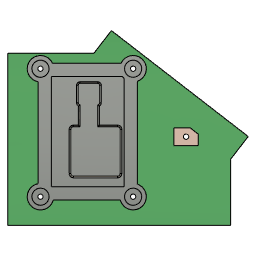
wiiWaterCooler_Base (Autodesk Fusion 360 design; units mm, degrees)
Autodesk Fusion 360 part; units mm, degrees
sketch "Wii" plane through (0, 0, 0) normal (0, 0, 1) x (1, 0, 0)
  line L0 (-39.75, -33.5) -> (61.25, -33.5)
  line L1 (-39.75, 44.5) -> (-39.75, -33.5)
  line L2 (-0.75, 44.5) -> (61.25, -3.5)
  line L3 (61.25, -33.5) -> (61.25, -3.5)
  line L4 (-39.75, 44.5) -> (-0.75, 44.5)
  circle A0 centre (-24.95, -20.5) radius 1.2
  circle A1 centre (-24.95, -20.5) radius 3.9
  circle A2 centre (41.05, 6.675) radius 1.2
  line L5 (14.5, -14.5) -> (-14.5, -14.5)
  line L6 (-14.5, -14.5) -> (-14.5, 14.5)
  line L7 (-14.5, 14.5) -> (14.5, 14.5)
  line L8 (14.5, 14.5) -> (14.5, -14.5)
  line L9 (14.5, -14.5) -> (-14.5, 14.5) construction
  line L10 (-14.5, -14.5) -> (14.5, 14.5) construction
  line L11 (4.5, 18.5) -> (-10.5, 18.5)
  line L12 (-10.5, 18.5) -> (-10.5, 33.5)
  line L13 (-10.5, 33.5) -> (4.5, 33.5)
  line L14 (4.5, 33.5) -> (4.5, 18.5)
  line L15 (4.5, 18.5) -> (-10.5, 33.5) construction
  line L16 (-10.5, 18.5) -> (4.5, 33.5) construction
  line L17 (10, 12.5) -> (-10, 12.5)
  line L18 (-12.5, 10) -> (-12.5, -10)
  line L19 (-10, -12.5) -> (10, -12.5)
  line L20 (12.5, -10) -> (12.5, 10)
  line L21 (12.5, 12.5) -> (-12.5, -12.5) construction
  line L22 (-12.5, 12.5) -> (12.5, -12.5) construction
  line L23 (1, 31.5) -> (-7, 31.5)
  line L24 (-8.5, 30) -> (-8.5, 22)
  line L25 (-7, 20.5) -> (1, 20.5)
  line L26 (2.5, 22) -> (2.5, 30)
  line L27 (2.5, 31.5) -> (-8.5, 20.5) construction
  line L28 (-8.5, 31.5) -> (2.5, 20.5) construction
  arc A3 (12.5, 10) -> (10, 12.5) centre (10, 10) ccw
  arc A4 (-10, 12.5) -> (-12.5, 10) centre (-10, 10) ccw
  arc A5 (-12.5, -10) -> (-10, -12.5) centre (-10, -10) ccw
  arc A6 (10, -12.5) -> (12.5, -10) centre (10, -10) ccw
  arc A7 (2.5, 30) -> (1, 31.5) centre (1, 30) ccw
  arc A8 (-7, 31.5) -> (-8.5, 30) centre (-7, 30) ccw
  arc A9 (-8.5, 22) -> (-7, 20.5) centre (-7, 22) ccw
  arc A10 (1, 20.5) -> (2.5, 22) centre (1, 22) ccw
  circle A11 centre (-24.95, 37.5) radius 1.2
  circle A12 centre (-24.95, 37.5) radius 3.9
  circle A13 centre (17.05, -20.5) radius 1.2
  circle A14 centre (17.05, -20.5) radius 3.9
  line L29 (42.9406, 10.675) -> (35.55, 10.675)
  line L30 (35.55, 10.675) -> (35.55, 2.675)
  line L31 (35.55, 2.675) -> (46.55, 2.675)
  line L32 (46.55, 2.675) -> (46.55, 7.8806)
  line L33 (44.6889, 9.3215) -> (35.55, 2.675) construction
  line L34 (35.55, 10.675) -> (46.55, 2.675) construction
  point P0 (-24.95, -20.5)
  point P1 (-3, 26)
  point P2 (41.05, 6.675)
  point P3 (-3, 26)
  point P4 (41.05, 6.675)
  dimension "d8" = 2.4
  dimension "d9" = 7.8
  dimension "d18" = 2.4
  dimension "d19" = 29
  dimension "d20" = 29
  dimension "d21" = 15
  dimension "d22" = 15
  dimension "d25" = 4
  dimension "d29" = 25
  dimension "d30" = 11
  dimension "d31" = 11
  dimension "d42" = 2.5
  dimension "d43" = 2.5
  dimension "d44" = 2.5
  dimension "d45" = 2.5
  dimension "d49" = 1.5
  dimension "d50" = 1.5
  dimension "d51" = 1.5
  dimension "d52" = 1.5
  dimension "d67" = 2.4
  dimension "d68" = 7.8
  dimension "d70" = 2.4
  dimension "d71" = 7.8
  constraint coincident P0 A0.centre
  constraint concentric A0 A1
  constraint perpendicular L5 L6
  constraint parallel L5 L7
  constraint parallel L6 L8
  constraint horizontal L5
  constraint coincident L9 origin
  constraint coincident L10 origin
  constraint perpendicular L11 L12
  constraint parallel L11 L13
  constraint parallel L12 L14
  constraint horizontal L11
  constraint coincident L15 P3
  constraint coincident L16 P3
  constraint coincident P4 P2
  constraint perpendicular L17 L18
  constraint parallel L17 L19
  constraint parallel L18 L20
  constraint horizontal L17
  constraint coincident L21 origin
  constraint coincident L22 origin
  constraint perpendicular L23 L24
  constraint parallel L23 L25
  constraint parallel L24 L26
  constraint horizontal L23
  constraint coincident L27 P3
  constraint coincident L28 P3
  constraint coincident P3 P1
  constraint tangent L20 A3
  constraint tangent L17 A3
  constraint tangent L18 A4
  constraint tangent L17 A4
  constraint coincident L21.end L19
  constraint coincident L21.end L18
  constraint tangent L19 A5
  constraint tangent L18 A5
  constraint coincident L22.end L19
  constraint coincident L22.end L20
  constraint tangent L19 A6
  constraint tangent L20 A6
  constraint tangent L26 A7
  constraint tangent L23 A7
  constraint coincident L28.start L24
  constraint coincident L28.start L23
  constraint tangent L24 A8
  constraint tangent L23 A8
  constraint coincident L27.end L25
  constraint coincident L27.end L24
  constraint tangent L25 A9
  constraint tangent L24 A9
  constraint coincident L28.end L25
  constraint coincident L28.end L26
  constraint tangent L25 A10
  constraint tangent L26 A10
  constraint concentric A11 A12
  constraint concentric A13 A14
  constraint perpendicular L29 L30
  constraint parallel L29 L31
  constraint parallel L30 L32
  constraint horizontal L29
  constraint coincident L33 P4
  constraint coincident L34 P4
  constraint coincident L2 L32.end
  constraint coincident L2 L33.start
  constraint coincident L2 L29.start
  measures "d8" diameter of A0
  measures "d9" diameter of A1
  measures "d18" diameter of A2
  measures "d19" distance of L6.end L7.end
  measures "d20" distance of L5.end L6.end
  measures "d21" distance of L12.end L13.end
  measures "d22" distance of L11.end L12.end
  measures "d25" distance of L7 L11
  measures "d29" distance of L21.end L22.end
  measures "d30" distance of L28.start L27.end
  measures "d31" distance of L27.end L28.end
  measures "d42" radius of A3
  measures "d43" radius of A4
  measures "d44" radius of A5
  measures "d45" radius of A6
  measures "d49" radius of A7
  measures "d50" radius of A8
  measures "d51" radius of A9
  measures "d52" radius of A10
  measures "d67" diameter of A11
  measures "d68" diameter of A12
  measures "d70" diameter of A13
  measures "d71" diameter of A14
extrude "Extrude14" add sketch "Wii" along normal blind 1.35 contours L2 L29 L30 L31 L32 | A1 | A12 | A14 makes body 1 at (-21.969, -20.7534, 0) makes body 2 at (20.031, -20.7534, 0) makes body 3 at (-21.969, 37.2466, 0) makes body 4 at (36.9833, 6.675, 0)
extrude "Extrude15" add sketch "Wii" along normal blind 1.35 separate body contours L0 L1 L2 L3 L4 L29 L30 L31 L32 | L5 L6 L7 L8 | L11 L12 L13 L14 | L17 L18 L19 L20 A3 A4 A5 A6 | L23 L24 L25 L26 A7 A8 A9 A10 makes body 5
extrude "Extrude16" add sketch "Wii" along normal blind 2 from surface at 1.35 separate body contours L5 L6 L7 L8 makes body 6
extrude "Extrude17" add sketch "Wii" along normal blind 2.75 from surface at 1.35 separate body contours L17 L18 L19 L20 A3 A4 A5 A6 makes body 7
combine "Combine4" operation add target body 7 tool bodies 6
fillet "Fillet3" radius 1.5 8 edges at (0, 12.5, 4.1) (-11.7678, 11.7678, 4.1) (-12.5, 0, 4.1) (-11.7678, -11.7678, 4.1) (0, -12.5, 4.1) (11.7678, -11.7678, 4.1) (12.5, 0, 4.1) (11.7678, 11.7678, 4.1) on bodies 7
extrude "Extrude18" add sketch "Wii" along normal blind 1.9 from surface at 1.35 separate body contours L11 L12 L13 L14 makes body 8
extrude "Extrude19" add sketch "Wii" along normal blind 2.65 from surface at 1.35 separate body contours L23 L24 L25 L26 A7 A8 A9 A10 makes body 9
combine "Combine5" operation add target body 9 tool bodies 8
fillet "Fillet4" radius 0.65 8 edges at (-3, 31.5, 4) (-8.0607, 31.0607, 4) (-8.5, 26, 4) (-8.0607, 20.9393, 4) (-3, 20.5, 4) (2.0607, 20.9393, 4) (2.5, 26, 4) (2.0607, 31.0607, 4) on bodies 9
copy_body "CopyPasteBodies1" bodies 1 makes body 10
move_body "Move1" bodies 10 to x (1, 0, 0) y (0, 1, 0) z (0, 0, 1) at (44, 58, 0)
move_body "Move3" bodies 10 to x (1, 0, 0) y (0, 1, 0) z (0, 0, 1) at (-2, 0, 0)
extrude "Extrude20" add 2 faces at (13.8135, 33.225, 0.45) (51.45, 4.0871, 0.9) along direction (0.612173, 0.790724, 0) blind 13 on bodies 5 bodies 5
extrude "Extrude21" add 1 faces at (45.5934, 14.1015, 0.45) along direction (0.790724, -0.612173, 0) blind 5 on bodies 5 bodies 5
sketch "Sketch2" plane through (0, 0, 1.35) normal (0, 0, 1) x (1, 0, 0)
  line L0 (46.55, 7.8806) -> (46.55, 2.675)
  line L1 (46.55, 2.675) -> (35.55, 2.675)
  line L2 (35.55, 2.675) -> (35.55, 10.675)
  line L3 (35.55, 10.675) -> (42.9406, 10.675)
  line L4 (42.9406, 10.675) -> (46.55, 7.8806)
  line L5 (69.2083, 6.7794) -> (7.2083, 54.7794)
  line L6 (7.2083, 54.7794) -> (-0.75, 44.5)
  line L7 (-0.75, 44.5) -> (-39.75, 44.5)
  line L8 (-39.75, 44.5) -> (-39.75, -33.5)
  line L9 (-39.75, -33.5) -> (61.25, -33.5)
  line L10 (61.25, -33.5) -> (61.25, -3.5)
  line L11 (61.25, -3.5) -> (69.2083, 6.7794)
  circle A0 centre (-24.95, 37.5) radius 3.9
  circle A1 centre (-24.95, -20.5) radius 3.9
  circle A2 centre (17.05, -20.5) radius 3.9
  circle A3 centre (17.05, 37.5) radius 1.1931
sketch "Sketch3" plane through (0, 0, 1.35) normal (0, 0, 1) x (1, 0, 0)
  circle A0 centre (17.05, 37.5) radius 3.8694
extrude "Extrude22" cut sketch "Sketch3" against normal blind 2 bodies 5
sketch "Sketch4" plane through (0, 0, 0) normal (0, 0, 1) x (1, 0, 0)
sketch "GPUcontact" plane through (0, 0, 4.1) normal (0, 0, 1) x (1, 0, 0)
  line L0 (11.201, -10) -> (11.201, 10)
  arc A0 (11.201, 10) -> (10, 11.201) centre (10, 10) ccw
  line L1 (10, 11.201) -> (-10, 11.201)
  arc A1 (-10, 11.201) -> (-11.201, 10) centre (-10, 10) ccw
  line L2 (-11.201, 10) -> (-11.201, -10)
  arc A2 (-11.201, -10) -> (-10, -11.201) centre (-10, -10) ccw
  line L3 (-10, -11.201) -> (10, -11.201)
  arc A3 (10, -11.201) -> (11.201, -10) centre (10, -10) ccw
sketch "CPUcontact" plane through (0, 0, 4) normal (0, 0, 1) x (1, 0, 0)
  line L0 (1, 30.85) -> (-7, 30.85)
  arc A0 (-7, 30.85) -> (-7.85, 30) centre (-7, 30) ccw
  line L1 (-7.85, 30) -> (-7.85, 22)
  arc A1 (-7.85, 22) -> (-7, 21.15) centre (-7, 22) ccw
  line L2 (-7, 21.15) -> (1, 21.15)
  arc A2 (1, 21.15) -> (1.85, 22) centre (1, 22) ccw
  line L3 (1.85, 22) -> (1.85, 30)
  arc A3 (1.85, 30) -> (1, 30.85) centre (1, 30) ccw
sketch "screwPost" plane through (0, 0, 1.35) normal (0, 0, 1) x (1, 0, 0)
  circle A0 centre (-24.95, 37.5) radius 1.2
  circle A1 centre (-24.95, 37.5) radius 3.9
extrude "Extrude23" add sketch "screwPost" 3 faces at (20.031, 37.2466, 1.35) (20.031, -20.7534, 1.35) (-21.969, -20.7534, 1.35) along normal blind 2.75 separate body on bodies 1 2 10 makes body 11 at (20.9452, -20.6944, 3.1833) makes body 12 at (-21.0548, 37.3056, 3.1833) makes body 13 at (20.9452, 37.3056, 3.1833) makes body 14 at (-21.0548, -20.6944, 3.1833)
extrude "Extrude24" add sketch "GPUcontact" along normal blind 3 separate body makes body 15
extrude "Extrude25" add sketch "CPUcontact" along normal blind 3.1 separate body makes body 16
extrude "Extrude26" add 4 faces at (-21.969, 37.2466, 4.1) (20.031, 37.2466, 4.1) (-21.969, -20.7534, 4.1) (20.031, -20.7534, 4.1) along direction (0, 0, 1) blind 3 on bodies 11 12 13 14 bodies 12 11 13 14
sketch "Sketch12" plane through (0, 0, 7.1) normal (0, 0, 1) x (1, 0, 0)
  circle A0 centre (-24.95, -20.5) radius 1.2
  circle A1 centre (-24.95, -20.5) radius 3.9
  line L0 (-24, -19) -> (16, -19)
  line L1 (16, -19) -> (16, 36)
  line L2 (16, 36) -> (-24, 36)
  line L3 (-24, 36) -> (-24, -19)
  line L4 (-20, -16) -> (13, -16)
  line L5 (13, -16) -> (13, 34)
  line L6 (13, 34) -> (-20, 34)
  line L7 (-20, 34) -> (-20, -16)
  constraint horizontal L0
  constraint vertical L1
  constraint horizontal L2
  constraint vertical L3
  constraint horizontal L4
  constraint vertical L5
  constraint horizontal L6
  constraint vertical L7
extrude "Extrude27" add sketch "Sketch12" along normal blind 2 separate body contours A1 L0 L3 | A1 L0 L1 L2 L3 picked at (-23.2156, -17.8274) makes body 17
sketch "Sketch14" plane through (0, 0, 7.1) normal (0, 0, 1) x (1, 0, 0)
  arc A0 (10, -11.201) -> (11.201, -10) centre (10, -10) ccw
  line L0 (11.201, -10) -> (11.201, 10)
  arc A1 (11.201, 10) -> (10, 11.201) centre (10, 10) ccw
  line L1 (10, 11.201) -> (-10, 11.201)
  arc A2 (-10, 11.201) -> (-11.201, 10) centre (-10, 10) ccw
  line L2 (-11.201, 10) -> (-11.201, -10)
  arc A3 (-11.201, -10) -> (-10, -11.201) centre (-10, -10) ccw
  line L3 (-10, -11.201) -> (10, -11.201)
  line L4 (-7, 30.85) -> (13, 30.85)
  line L5 (13, 30.85) -> (13, 34)
  line L6 (13, 34) -> (-7, 34)
  line L7 (-7, 34) -> (-7, 30.85)
  line L8 (-7, 30.85) -> (-20, 30.85)
  line L9 (-20, 30.85) -> (-20, 34)
  line L10 (-20, 34) -> (-7, 34)
  line L11 (-7, 34) -> (-7, 30.85)
  line L12 (-7.85, 30) -> (-20, 30)
  line L13 (-20, 30) -> (-20, 30.85)
  line L14 (-20, 30.85) -> (-7.85, 30.85)
  line L15 (-7.85, 30.85) -> (-7.85, 30)
  line L16 (-7.85, 30) -> (-20, 30)
  line L17 (-20, 30) -> (-20, 12.5)
  line L18 (-20, 12.5) -> (-7.85, 12.5)
  line L19 (-7.85, 12.5) -> (-7.85, 30)
  line L20 (-7, 21.15) -> (-7.85, 21.15)
  line L21 (-7.85, 21.15) -> (-7.85, 12.5)
  line L22 (-7.85, 12.5) -> (-7, 12.5)
  line L23 (-7, 12.5) -> (-7, 21.15)
  line L24 (-7, 12.5) -> (1, 12.5)
  line L25 (1, 12.5) -> (1, 21.15)
  line L26 (1, 21.15) -> (-7, 21.15)
  line L27 (-7, 21.15) -> (-7, 12.5)
  line L28 (1.85, 22) -> (13, 22)
  line L29 (13, 22) -> (13, 30.85)
  line L30 (13, 30.85) -> (1.85, 30.85)
  line L31 (1.85, 30.85) -> (1.85, 22)
  line L32 (1, 21.15) -> (13, 21.15)
  line L33 (13, 21.15) -> (13, 12.5)
  line L34 (13, 12.5) -> (1, 12.5)
  line L35 (1, 12.5) -> (1, 21.15)
  line L36 (1.85, 22) -> (13, 22)
  line L37 (13, 22) -> (13, 21.15)
  line L38 (13, 21.15) -> (1.85, 21.15)
  line L39 (1.85, 21.15) -> (1.85, 22)
  line L40 (-10, 11.201) -> (10, 11.201)
  line L41 (10, 11.201) -> (10, 12.5)
  line L42 (10, 12.5) -> (-10, 12.5)
  line L43 (-10, 12.5) -> (-10, 11.201)
  line L44 (-11.201, 10) -> (-20, 10)
  line L45 (-20, 10) -> (-20, 12.5)
  line L46 (-20, 12.5) -> (-11.201, 12.5)
  line L47 (-11.201, 12.5) -> (-11.201, 10)
  line L48 (-10, 11.201) -> (-11.201, 11.201)
  line L49 (-11.201, 11.201) -> (-11.201, 12.5)
  line L50 (-11.201, 12.5) -> (-10, 12.5)
  line L51 (-10, 12.5) -> (-10, 11.201)
  line L52 (11.201, 10) -> (13, 10)
  line L53 (13, 10) -> (13, 12.5)
  line L54 (13, 12.5) -> (11.201, 12.5)
  line L55 (11.201, 12.5) -> (11.201, 10)
  line L56 (10, 11.201) -> (11.201, 11.201)
  line L57 (11.201, 11.201) -> (11.201, 12.5)
  line L58 (11.201, 12.5) -> (10, 12.5)
  line L59 (10, 12.5) -> (10, 11.201)
  line L60 (11.201, 10) -> (13, 10)
  line L61 (13, 10) -> (13, -10)
  line L62 (13, -10) -> (11.201, -10)
  line L63 (11.201, -10) -> (11.201, 10)
  line L64 (10, -11.201) -> (13, -11.201)
  line L65 (13, -11.201) -> (13, -16)
  line L66 (13, -16) -> (10, -16)
  line L67 (10, -16) -> (10, -11.201)
  line L68 (11.201, -10) -> (13, -10)
  line L69 (13, -10) -> (13, -11.201)
  line L70 (13, -11.201) -> (11.201, -11.201)
  line L71 (11.201, -11.201) -> (11.201, -10)
  line L72 (10, -11.201) -> (-20, -11.201)
  line L73 (-20, -11.201) -> (-20, -16)
  line L74 (-20, -16) -> (10, -16)
  line L75 (10, -16) -> (10, -11.201)
  line L76 (-11.201, -10) -> (-20, -10)
  line L77 (-20, -10) -> (-20, -11.201)
  line L78 (-20, -11.201) -> (-11.201, -11.201)
  line L79 (-11.201, -11.201) -> (-11.201, -10)
  line L80 (-11.201, -10) -> (-20, -10)
  line L81 (-20, -10) -> (-20, 10)
  line L82 (-20, 10) -> (-11.201, 10)
  line L83 (-11.201, 10) -> (-11.201, -10)
  constraint horizontal L4
  constraint vertical L5
  constraint horizontal L6
  constraint vertical L7
  constraint horizontal L8
  constraint vertical L9
  constraint horizontal L10
  constraint vertical L11
  constraint horizontal L12
  constraint vertical L13
  constraint horizontal L14
  constraint vertical L15
  constraint horizontal L16
  constraint vertical L17
  constraint horizontal L18
  constraint vertical L19
  constraint horizontal L20
  constraint vertical L21
  constraint horizontal L22
  constraint vertical L23
  constraint horizontal L24
  constraint vertical L25
  constraint horizontal L26
  constraint vertical L27
  constraint horizontal L28
  constraint vertical L29
  constraint horizontal L30
  constraint vertical L31
  constraint horizontal L32
  constraint vertical L33
  constraint horizontal L34
  constraint vertical L35
  constraint horizontal L36
  constraint vertical L37
  constraint horizontal L38
  constraint vertical L39
  constraint horizontal L40
  constraint vertical L41
  constraint horizontal L42
  constraint vertical L43
  constraint coincident L34 L41.end
  constraint coincident L1.end A2.start
  constraint horizontal L44
  constraint vertical L45
  constraint horizontal L46
  constraint vertical L47
  constraint coincident A2.end L2.start
  constraint horizontal L48
  constraint vertical L49
  constraint horizontal L50
  constraint vertical L51
  constraint horizontal L52
  constraint vertical L53
  constraint horizontal L54
  constraint vertical L55
  constraint coincident L0.end A1.start
  constraint horizontal L56
  constraint vertical L57
  constraint horizontal L58
  constraint vertical L59
  constraint coincident A1.end L1.start
  constraint horizontal L60
  constraint vertical L61
  constraint horizontal L62
  constraint vertical L63
  constraint horizontal L64
  constraint vertical L65
  constraint horizontal L66
  constraint vertical L67
  constraint coincident A0.start L3.end
  constraint horizontal L68
  constraint vertical L69
  constraint horizontal L70
  constraint vertical L71
  constraint horizontal L72
  constraint vertical L73
  constraint horizontal L74
  constraint vertical L75
  constraint horizontal L76
  constraint vertical L77
  constraint horizontal L78
  constraint vertical L79
  constraint coincident L2.end A3.start
  constraint horizontal L80
  constraint vertical L81
  constraint horizontal L82
  constraint vertical L83
extrude "Extrude28" add sketch "Sketch14" against normal blind 1 separate body contours L3 L67 L72 L73 L74 L75 L78 | A0 L64 L71 | L64 L65 L66 L67 L70 L75 | L0 L52 L60 L61 L62 L63 L68 | L62 L64 L68 L69 L70 L71 | A3 L72 L79 | L34 L52 L53 L54 L55 L57 L60 | A1 L55 L56 | L2 L44 L76 L80 L81 L82 L83 | L72 L76 L77 L78 L79 L80 | L1 L18 L22 L24 L34 L40 L41 L42 L43 L51 L59 | L34 L41 L55 L56 L57 L58 L59 | A2 L47 L48 | L18 L44 L45 L46 L47 L49 L82 | L18 L43 L47 L48 L49 L50 L51 | L25 L32 L33 L34 L35 L38 L42 L54 L58 | L12 L16 L17 L18 L19 L21 L42 L46 L50 | L23 L24 L25 L26 L27 L35 L42 | L28 L32 L36 L37 L38 L39 | L19 L20 L21 L22 L23 L27 L42 | L4 L28 L29 L30 L31 L36 | L8 L12 L13 L14 L15 L16 | L4 L5 L6 L7 L11 L30 | L7 L8 L9 L10 L11 L14 makes body 18
sketch "Sketch15" plane through (0, 0, 7.1) normal (0, 0, 1) x (1, 0, 0)
  arc A0 (1.85, 30) -> (1, 30.85) centre (1, 30) ccw
  line L0 (1, 30.85) -> (-7, 30.85)
  arc A1 (-7, 30.85) -> (-7.85, 30) centre (-7, 30) ccw
  line L1 (-7.85, 30) -> (-7.85, 22)
  arc A2 (-7.85, 22) -> (-7, 21.15) centre (-7, 22) ccw
  line L2 (-7, 21.15) -> (1, 21.15)
  arc A3 (1, 21.15) -> (1.85, 22) centre (1, 22) ccw
  line L3 (1.85, 22) -> (1.85, 30)
extrude "Extrude29" add 2 faces at (-7.85, 24.1, 6.7667) (-7.85, 30.5667, 6.7667) along direction (1, 0, 0) blind 1.1 on bodies 18 bodies 18 16
extrude "Extrude30" add 2 faces at (1.85, 21.7167, 6.4333) (1.85, 30.5667, 6.7667) along direction (-1, 0, 0) blind 1 on bodies 18 bodies 18
extrude "Extrude31" add 1 faces at (-22.6667, 17.7608, 7.1) along direction (0, 0, -1) blind 0.1 on bodies 17 bodies 17 11 12 13 14 18
extrude "Extrude32" add sketch "Sketch15" against normal blind 3.1 separate body makes body 19
extrude "Extrude33" cut 1 faces at (-4.6167, 24.6667, 7.1) along direction (0, 0, -1) blind 3.1 on bodies 19 bodies 17
extrude "Extrude34" cut 2 faces at (-2.933, 3.3333, 7.1) (-4.6167, 24.6667, 7.1) along direction (0, 0, -1) blind 1 on bodies 15 19 bodies 15 19
sketch "Sketch17" plane through (0, 0, 7.1) normal (0, 0, 1) x (1, 0, 0)
  arc A0 (1.85, 30) -> (1, 30.85) centre (1, 30) ccw
  line L0 (1.85, 30) -> (1.85, 22)
  arc A1 (1, 21.15) -> (1.85, 22) centre (1, 22) ccw
  line L1 (1, 21.15) -> (-7, 21.15)
  arc A2 (-7.85, 22) -> (-7, 21.15) centre (-7, 22) ccw
  line L2 (-7.85, 22) -> (-7.85, 30)
  arc A3 (-7, 30.85) -> (-7.85, 30) centre (-7, 30) ccw
  line L3 (-7, 30.85) -> (1, 30.85)
  arc A4 (-10, 11.201) -> (-11.201, 10) centre (-10, 10) ccw
  line L4 (-10, 11.201) -> (10, 11.201)
  arc A5 (11.201, 10) -> (10, 11.201) centre (10, 10) ccw
  line L5 (11.201, 10) -> (11.201, -10)
  arc A6 (10, -11.201) -> (11.201, -10) centre (10, -10) ccw
  line L6 (10, -11.201) -> (-10, -11.201)
  arc A7 (-11.201, -10) -> (-10, -11.201) centre (-10, -10) ccw
  line L7 (-11.201, -10) -> (-11.201, 10)
  line L8 (-20, 34) -> (-20, -16)
  line L9 (-20, -16) -> (13, -16)
  line L10 (13, -16) -> (13, 34)
  line L11 (13, 34) -> (-20, 34)
  line L12 (-7, 21.15) -> (1.0093, 21.15)
  line L13 (1.0093, 21.15) -> (1.0093, 11.201)
  line L14 (1.0093, 11.201) -> (-7, 11.201)
  line L15 (-7, 11.201) -> (-7, 21.15)
  constraint horizontal L12
  constraint vertical L13
  constraint horizontal L14
  constraint vertical L15
  constraint coincident L4 L13.end
  constraint coincident L1.end A2.end
extrude "Extrude35" cut sketch "Sketch17" against normal blind 1 contours A1 L1 L4 L12 L13 L14 L15 bodies 17
sketch "Sketch18" plane through (0, 0, 6.1) normal (0, 0, 1) x (1, 0, 0)
  arc A0 (10, -11.201) -> (11.201, -10) centre (10, -10) ccw
  line L0 (11.201, -10) -> (11.201, 10)
  arc A1 (11.201, 10) -> (10, 11.201) centre (10, 10) ccw
  line L1 (10, 11.201) -> (-10, 11.201)
  arc A2 (-10, 11.201) -> (-11.201, 10) centre (-10, 10) ccw
  line L2 (-11.201, 10) -> (-11.201, -10)
  arc A3 (-11.201, -10) -> (-10, -11.201) centre (-10, -10) ccw
  line L3 (-10, -11.201) -> (10, -11.201)
  line L4 (-6.9999, 11.201) -> (1, 11.201)
  line L5 (1, 11.201) -> (1, 21.15)
  line L6 (1, 21.15) -> (-6.9999, 21.15)
  line L7 (-6.9999, 21.15) -> (-6.9999, 11.201)
  constraint horizontal L4
  constraint vertical L5
  constraint horizontal L6
  constraint vertical L7
  constraint coincident L1 L4.start
extrude "Extrude36" add sketch "Sketch18" against normal blind 1 contours L1 L4 L5 L6 L7 bodies 15 17 19
extrude "Extrude37" add 1 faces at (-1.6666, 14.5173, 5.1) along direction (0, 0, -1) blind 1 on bodies 15 bodies 15
sketch "Sketch21" plane through (0, 0, 7.1) normal (0, 0, 1) x (1, 0, 0)
  line L0 (16, -19) -> (13.45, -19)
  arc A0 (13.45, -19) -> (16, -16.744) centre (17.05, -20.5) ccw
  line L1 (16, -16.744) -> (16, -19)
  circle A1 centre (17.05, -20.5) radius 1.2
  circle A2 centre (17.05, -20.5) radius 6
  dimension "d140" = 12
  constraint concentric A0 A2
  measures "d140" diameter of A2
sketch "Sketch22" plane through (0, 0, 7.1) normal (0, 0, 1) x (1, 0, 0)
  line L0 (-24, -19) -> (-24, -16.7175)
  arc A0 (-24, -16.7175) -> (-21.35, -19) centre (-24.95, -20.5) ccw
  line L1 (-21.35, -19) -> (-24, -19)
  circle A1 centre (-24.95, -20.5) radius 1.2
  circle A2 centre (-24.95, -20.5) radius 6
  dimension "d141" = 12
  constraint concentric A0 A2
  measures "d141" diameter of A2
sketch "Sketch23" plane through (0, 0, 7.1) normal (0, 0, 1) x (1, 0, 0)
  line L0 (-24, 36) -> (-21.35, 36)
  arc A0 (-21.35, 36) -> (-24, 33.7175) centre (-24.95, 37.5) ccw
  line L1 (-24, 33.7175) -> (-24, 36)
  circle A1 centre (-24.95, 37.5) radius 1.2
  circle A2 centre (-24.95, 37.5) radius 6
  dimension "d142" = 12
  constraint concentric A0 A2
  measures "d142" diameter of A2
sketch "Sketch24" plane through (0, 0, 7.1) normal (0, 0, 1) x (1, 0, 0)
  line L0 (13.45, 36) -> (16, 36)
  line L1 (16, 36) -> (16, 33.744)
  arc A0 (16, 33.744) -> (13.45, 36) centre (17.05, 37.5) ccw
  circle A1 centre (17.05, 37.5) radius 1.2
  circle A2 centre (17.05, 37.5) radius 6
  dimension "d143" = 12
  constraint concentric A0 A2
  measures "d143" diameter of A2
extrude "Extrude38" add sketch "Sketch23" sketch "Sketch24" sketch "Sketch22" sketch "Sketch21" along normal blind 2 contours A2 of sketch 2 contours A2 of sketch 3 contours A2 of sketch 4 contours A2 bodies 15
sketch "Sketch25" plane through (0, 0, 7.1) normal (0, 0, 1) x (1, 0, 0)
  line L0 (16, -19) -> (13.45, -19)
  arc A0 (13.45, -19) -> (16, -16.744) centre (17.05, -20.5) ccw
  line L1 (16, -16.744) -> (16, -19)
  circle A1 centre (17.05, -20.5) radius 1.2
  circle A2 centre (17.05, -20.5) radius 3.9
  constraint concentric A0 A2
sketch "Sketch26" plane through (0, 0, 7.1) normal (0, 0, 1) x (1, 0, 0)
  line L0 (-24, 36) -> (-21.35, 36)
  arc A0 (-21.35, 36) -> (-24, 33.7175) centre (-24.95, 37.5) ccw
  line L1 (-24, 33.7175) -> (-24, 36)
  circle A1 centre (-24.95, 37.5) radius 1.2
  circle A2 centre (-24.95, 37.5) radius 3.8668
  constraint concentric A0 A2
sketch "Sketch27" plane through (0, 0, 7.1) normal (0, 0, 1) x (1, 0, 0)
  line L0 (13.45, 36) -> (16, 36)
  line L1 (16, 36) -> (16, 33.744)
  arc A0 (16, 33.744) -> (13.45, 36) centre (17.05, 37.5) ccw
  circle A1 centre (17.05, 37.5) radius 1.2
  circle A2 centre (17.05, 37.5) radius 3.9
  constraint concentric A0 A2
sketch "Sketch28" plane through (0, 0, 7.1) normal (0, 0, 1) x (1, 0, 0)
  line L0 (-24, -19) -> (-24, -16.7175)
  arc A0 (-24, -16.7175) -> (-21.35, -19) centre (-24.95, -20.5) ccw
  line L1 (-21.35, -19) -> (-24, -19)
  circle A1 centre (-24.95, -20.5) radius 1.2
  circle A2 centre (-24.95, -20.5) radius 3.9
  constraint concentric A0 A2
extrude "Extrude39" cut sketch "Sketch26" sketch "Sketch25" sketch "Sketch27" sketch "Sketch28" along normal blind 25 contours L0 L1 A2 | L0 L1 A2 of sketch 2 of sketch 3 of sketch 4 bodies 15
extrude "Extrude40" add 1 faces at (1.1135, -19, 8.4333) along direction (0, -1, 0) blind 3 on bodies 15 bodies 15
extrude "Extrude41" add 1 faces at (16, 0.8025, 8.4333) along direction (1, 0, 0) blind 2 on bodies 15 bodies 15
extrude "Extrude42" add 1 faces at (-9.0135, 36, 7.7667) along direction (0, 1, 0) blind 3 on bodies 15 bodies 15
extrude "Extrude43" add 1 faces at (-24, 16.1919, 8.4333) along direction (-1, 0, 0) blind 2 on bodies 15 bodies 15
fillet "Fillet5" radius 0.75 18 edges at (-7.601, 21.399, 7.1) (-7.85, 26, 7.1) (-7.601, 30.601, 7.1) (-3, 30.85, 7.1) (1.601, 30.601, 7.1) (1.85, 26, 7.1) (1.601, 21.399, 7.1) (1.0093, 16.1755, 7.1) (-7, 16.1755, 7.1) (5.5047, 11.201, 7.1) (10.8492, 10.8492, 7.1) (11.201, 0, 7.1) (10.8492, -10.8492, 7.1) (0, -11.201, 7.1) (-10.8492, -10.8492, 7.1) (-11.201, 0, 7.1) (-10.8492, 10.8492, 7.1) (-8.5, 11.201, 7.1) on bodies 15
extrude "Extrude44" add 1 faces at (-9.0135, 39, 7.7667) along direction (0, 1, 0) blind 1 on bodies 15 bodies 15
extrude "Extrude45" add 1 faces at (11.4313, 39.8913, 7.1) along direction (0, 0, 1) blind 2 on bodies 15 bodies 15
extrude "Extrude46" add 1 faces at (-19.3313, 39.8913, 7.1) along direction (0, 0, 1) blind 2 on bodies 15 bodies 15
extrude "Extrude47" add 1 faces at (-25.9889, 31.585, 7.1) along direction (0, 0, 1) blind 2 on bodies 15 bodies 15
extrude "Extrude48" add 1 faces at (-25.9889, -14.585, 7.1) along direction (0, 0, 1) blind 2 on bodies 15 bodies 15
extrude "Extrude49" add 1 faces at (18, 0.8081, 7.7667) along direction (1, 0, 0) blind 1 on bodies 15 bodies 15
extrude "Extrude50" add 1 faces at (18.8905, 31.7082, 7.1) along direction (0, 0, 1) blind 2 on bodies 15 bodies 15
extrude "Extrude51" add 1 faces at (18.8905, -14.7082, 7.1) along direction (0, 0, 1) blind 2 on bodies 15 bodies 15
sketch "Sketch16" plane through (0, 0, 7.1) normal (0, 0, 1) x (1, 0, 0)
  arc A0 (10, -11.201) -> (11.201, -10) centre (10, -10) ccw
  line L0 (11.201, -10) -> (11.201, 10)
  arc A1 (11.201, 10) -> (10, 11.201) centre (10, 10) ccw
  line L1 (10, 11.201) -> (-10, 11.201)
  arc A2 (-10, 11.201) -> (-11.201, 10) centre (-10, 10) ccw
  line L2 (-11.201, 10) -> (-11.201, -10)
  arc A3 (-11.201, -10) -> (-10, -11.201) centre (-10, -10) ccw
  line L3 (-10, -11.201) -> (10, -11.201)
  line L4 (-9, -10.5) -> (-6, -10.5)
  line L5 (-6, -10.5) -> (-6, 9.5)
  line L6 (-6, 9.5) -> (-9, 9.5)
  line L7 (-9, 9.5) -> (-9, -10.5)
  line L8 (-5, 9.5) -> (-5, -10.5)
  line L9 (-5, -10.5) -> (-2, -10.5)
  line L10 (-2, -10.5) -> (-2, 9.5)
  line L11 (-2, 9.5) -> (-5, 9.5)
  line L12 (2, -10.5) -> (2, 9.5)
  line L13 (-1, 9.5) -> (-1, -10.5)
  line L14 (-1, -10.5) -> (2, -10.5)
  line L15 (2, 9.5) -> (-1, 9.5)
  line L16 (6, 9.5) -> (3, 9.5)
  line L17 (3, 9.5) -> (3, -10.5)
  line L18 (6, -10.5) -> (6, 9.5)
  line L19 (3, -10.5) -> (6, -10.5)
  line L20 (10, -10.5) -> (10, 9.5)
  line L21 (7, 9.5) -> (7, -10.5)
  line L22 (7, -10.5) -> (10, -10.5)
  line L23 (10, 9.5) -> (7, 9.5)
  dimension "d122" = 3
  dimension "d123" = 20
  dimension "d124" = 3
  dimension "d125" = 20
  dimension "d126" = 3
  dimension "d127" = 20
  dimension "d128" = 3
  dimension "d129" = 20
  dimension "d130" = 3
  dimension "d131" = 20
  constraint horizontal L4
  constraint vertical L5
  constraint horizontal L6
  constraint vertical L7
  constraint horizontal L9
  constraint vertical L10
  constraint horizontal L11
  constraint vertical L8
  constraint horizontal L14
  constraint vertical L12
  constraint horizontal L15
  constraint vertical L13
  constraint horizontal L19
  constraint vertical L18
  constraint horizontal L16
  constraint vertical L17
  constraint horizontal L22
  constraint vertical L20
  constraint horizontal L23
  constraint vertical L21
  measures "d122" distance of L4.start L4.end
  measures "d123" distance of L4.start L6.end
  measures "d124" distance of L9.end L8.end
  measures "d125" distance of L8.start L8.end
  measures "d126" distance of L12.start L13.end
  measures "d127" distance of L13.start L13.end
  measures "d128" distance of L17.end L18.start
  measures "d129" distance of L16.end L17.end
  measures "d130" distance of L21.end L20.start
  measures "d131" distance of L21.end L21.start
sketch "Sketch13" plane through (0, 0, 7.1) normal (0, 0, 1) x (1, 0, 0)
  arc A0 (10, -11.201) -> (11.201, -10) centre (10, -10) ccw
  line L0 (11.201, -10) -> (11.201, 10)
  arc A1 (11.201, 10) -> (10, 11.201) centre (10, 10) ccw
  line L1 (10, 11.201) -> (-10, 11.201)
  arc A2 (-10, 11.201) -> (-11.201, 10) centre (-10, 10) ccw
  line L2 (-11.201, 10) -> (-11.201, -10)
  arc A3 (-11.201, -10) -> (-10, -11.201) centre (-10, -10) ccw
  line L3 (-10, -11.201) -> (10, -11.201)
  line L4 (-20, -16) -> (-11.201, -16)
  line L5 (-11.201, -16) -> (-11.201, 10)
  line L6 (-11.201, 10) -> (-20, 10)
  line L7 (-20, 10) -> (-20, -16)
  line L8 (-11.201, 10) -> (-20, 10)
  line L9 (-20, 10) -> (-20, 34)
  line L10 (-20, 34) -> (-11.201, 34)
  line L11 (-11.201, 34) -> (-11.201, 10)
  line L12 (-11.201, 34) -> (-7.85, 34)
  line L13 (-7.85, 34) -> (-7.85, 22)
  line L14 (-7.85, 22) -> (-11.201, 22)
  line L15 (-11.201, 22) -> (-11.201, 34)
  line L16 (-7.85, 22) -> (-11.201, 22)
  line L17 (-11.201, 22) -> (-11.201, 11.2021)
  line L18 (-11.201, 11.2021) -> (-7.85, 11.2021)
  line L19 (-7.85, 11.2021) -> (-7.85, 22)
  constraint horizontal L4
  constraint vertical L5
  constraint horizontal L6
  constraint vertical L7
  constraint coincident A2.end L2.start
  constraint horizontal L8
  constraint vertical L9
  constraint horizontal L10
  constraint vertical L11
  constraint horizontal L12
  constraint vertical L13
  constraint horizontal L14
  constraint vertical L15
  constraint horizontal L16
  constraint vertical L17
  constraint horizontal L18
  constraint vertical L19
  constraint coincident L11 L17.end
sketch "Sketch8" plane through (0, 0, 4) normal (0, 0, 1) x (1, 0, 0)
named bodies: "screwHole 1", "screwHole 2", "screwHole 3", "screwHole 5", "PCB", "GPU", "CPU", "Screw Hole 1", "screwHole 4", "GPUContact", "CPUContact", "blockBottom", "CPUcontact"
